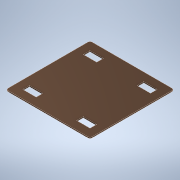
# Autodesk Inventor part: RobotBase
Saved by Autodesk Inventor 2022.3 (Build 263350000, 350)
## iProperties
Created: 2022-04-28
Part Number: RobotBase
Material: Bronze, Cast
Document SubType Name: Modeling
Designer: Robert Nies
Density: 8.87 g/cm^3
Appearance: Bronze - Satin
Author: Robert Nies
Autodesk Inventor part; units mm, degrees
ref_plane "YZ Plane" through (0, 0, 0) normal (1, 0, 0) x (0, 1, 0)
ref_plane "XZ Plane" through (0, 0, 0) normal (0, 1, 0) x (-1, 0, 0)
ref_plane "XY Plane" through (0, 0, 0) normal (0, 0, 1) x (1, 0, 0)
sketch "Sketch1" plane through (0, 0, 0) normal (0, 1, 0) x (-1, 0, 0)
  line L0 (0, 0) -> (-254, 0)
  line L1 (-254, 0) -> (-254, -254)
  line L2 (-254, -254) -> (0, -254)
  line L3 (0, -254) -> (0, 0)
  dimension "d0" = 254
  dimension "d1" = 254
  constraints: 8 end point, 2 parallel, 1 horizontal, 1 perpendicular
  measures "d0" distance of L2.end L1.end
  measures "d1" distance of L1.end L0.end
extrude "Extrusion1" add sketch "Sketch1" along normal blind 3.175
fillet "Fillet1" radius 6.35 4 edges at (0, 1.5875, 0) (254, 1.5875, 0) (254, 1.5875, -254) (0, 1.5875, -254)
sketch "Sketch2" plane through (0, 3.175, 0) normal (0, 1, 0) x (1, 0, 0)
  line L0 (25.4, 228.6) -> (66.04, 228.6)
  line L1 (66.04, 228.6) -> (66.04, 208.28)
  line L2 (66.04, 208.28) -> (25.4, 208.28)
  line L3 (25.4, 208.28) -> (25.4, 228.6)
  line L4 (247.65, 254) -> (6.35, 254) projected
  line L5 (0, 247.65) -> (0, 6.35) projected
  line L6 (187.96, 228.6) -> (228.6, 228.6)
  line L7 (228.6, 228.6) -> (228.6, 208.28)
  line L8 (228.6, 208.28) -> (187.96, 208.28)
  line L9 (187.96, 208.28) -> (187.96, 228.6)
  line L10 (25.4, 45.72) -> (66.04, 45.72)
  line L11 (66.04, 45.72) -> (66.04, 25.4)
  line L12 (66.04, 25.4) -> (25.4, 25.4)
  line L13 (25.4, 25.4) -> (25.4, 45.72)
  line L14 (187.96, 45.72) -> (228.6, 45.72)
  line L15 (228.6, 45.72) -> (228.6, 25.4)
  line L16 (228.6, 25.4) -> (187.96, 25.4)
  line L17 (187.96, 25.4) -> (187.96, 45.72)
  line L18 (254, 6.35) -> (254, 247.65) projected
  line L19 (6.35, 0) -> (247.65, 0) projected
  point P0 (0, 0)
  point P1 (45.72, 228.6)
  point P2 (228.6, 218.44)
  point P3 (45.72, 25.4)
  point P4 (25.4, 35.56)
  point P5 (228.6, 35.56)
  dimension "d5" = 40.64
  dimension "d6" = 20.32
  dimension "d7" = 25.4
  dimension "d8" = 25.4
  dimension "d11" = 20.32
  dimension "d12" = 40.64
  dimension "d13" = 40.64
  dimension "d14" = 20.32
  dimension "d15" = 40.64
  dimension "d16" = 20.32
  dimension "d17" = 25.4
  dimension "d18" = 25.4
  dimension "d19" = 25.4
  dimension "d20" = 25.4
  dimension "d21" = 25.4
  dimension "d22" = 25.4
  constraints: 32 end point, 8 parallel, 5 midpoint, 4 horizontal, 4 perpendicular
  measures "d5" distance of L1.end L2.end
  measures "d6" distance of L0.end L1.end
  measures "d7" distance from line of L4 point (45.72, 228.6)
  measures "d8" distance from line of L5 L0.start
  measures "d11" distance of L6.end L7.end
  measures "d12" distance of L7.end L8.end
  measures "d13" distance of L11.end L12.end
  measures "d14" distance of L10.end L11.end
  measures "d15" distance of L15.end L16.end
  measures "d16" distance of L14.end L15.end
  measures "d17" distance between parallel lines of L4 L6
  measures "d18" distance from line of L18 point (228.6, 218.44)
  measures "d19" distance from line of L19 point (45.72, 25.4)
  measures "d20" distance from line of L5 point (25.4, 35.56)
  measures "d21" distance from line of L18 point (228.6, 35.56)
  measures "d22" distance between parallel lines of L19 L16
extrude "Extrusion2" cut sketch "Sketch2" against normal blind 3.175
equation "\"d11\" = d6"
equation "\"d12\" = d5"
equation "\"d13\" = d5"
equation "\"d14\" = d6"
equation "\"d15\" = d5"
equation "\"d16\" = d6"
equation "\"d17\" = d7"
equation "\"d20\" = d8"
equation "\"d21\" = d18"
equation "\"d22\" = d19"
body "Solid1"
